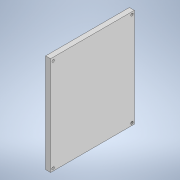
# Autodesk Inventor part: weather_side
Saved by Autodesk Inventor 2021 (Build 250183000, 183)
## iProperties
Created: 2020-04-05
Part Number: weather_side
Material: Generic
Document SubType Name: Modeling
Designer: Daniel
Density: 1 g/cm^3
Appearance: Default
Author: Daniel
Autodesk Inventor part; units mm, degrees
ref_plane "YZ Plane" through (0, 0, 0) normal (1, 0, 0) x (0, 1, 0)
ref_plane "XZ Plane" through (0, 0, 0) normal (0, 1, 0) x (-1, 0, 0)
ref_plane "XY Plane" through (0, 0, 0) normal (0, 0, 1) x (1, 0, 0)
sketch "Sketch1" plane through (0, 0, 0) normal (1, 0, 0) x (0, 1, 0)
  line L0 (0, 0) -> (100, 0)
  line L1 (100, 0) -> (100, -85)
  line L2 (100, -85) -> (0, -85)
  line L3 (0, -85) -> (0, 0)
  dimension "d0" = 100
  dimension "d1" = 85
  dimension "d2" = 100
  constraints: 8 end point, 2 perpendicular, 1 horizontal
  measures "d0" distance of L0.start L0.end
  measures "d1" distance of L0.end L1.end
  measures "d2" distance of L1.end L2.end
extrude "Extrusion1" add sketch "Sketch1" along normal blind 5
sketch "Sketch2" plane through (5, 0, 0) normal (1, 0, 0) x (0, 0, -1)
  line L0 (3.7344, 0) -> (1.2344, 0) construction
  line L1 (0, 0) -> (85, 0) construction
  line L2 (1.2344, 0) -> (1.2344, 2.5) construction
  line L3 (0, 100) -> (0, 0) construction
  line L4 (0, 3.0654) -> (0, 5.5654) construction
  line L5 (0, 5.5654) -> (2.5, 5.5654) construction
  circle A0 centre (2.5, 2.5) radius 1.255
  line L6 (79.4667, 0) -> (79.4667, 2.5) construction
  line L7 (85, 0) -> (85, 100) construction
  line L8 (85, 3.0654) -> (85, 0.5654) construction
  line L9 (85, 0.5654) -> (82.5, 0.5654) construction
  circle A1 centre (82.5, 2.5) radius 1.255 construction
  circle A2 centre (82.5, 2.5) radius 1.255
  line L10 (85, 97.4626) -> (82.5, 97.4626) construction
  line L11 (85, 100) -> (0, 100) construction
  line L12 (81.6079, 100) -> (84.1079, 100) construction
  line L13 (84.1079, 100) -> (84.1079, 97.5) construction
  circle A3 centre (82.5, 97.5) radius 1.25 construction
  circle A4 centre (82.5, 97.5) radius 1.255
  line L14 (0, 96.7939) -> (2.5, 96.7939) construction
  line L15 (2.6492, 100) -> (2.6492, 97.5) construction
  circle A5 centre (2.6492, 96.7939) radius 1.255
  dimension "d5" = 2.5
  dimension "d6" = 2.5
  dimension "d7" = 2.5
  dimension "d8" = 2.5
  dimension "d9" = 2.51
  dimension "d10" = 2.5
  dimension "d11" = 2.5
  dimension "d12" = 2.5
  dimension "d13" = 2.51
  dimension "d14" = 2.51
  dimension "d15" = 2.5
  dimension "d16" = 2.5
  dimension "d17" = 2.5
  dimension "d18" = 2.5
  dimension "d19" = 2.51
  dimension "d20" = 2.5
  dimension "d21" = 2.5
  dimension "d22" = 2.51
  constraints: 24 end point, 11 point on line, 7 perpendicular, 6 centre point, 2 coincident, 1 horizontal
  measures "d5" distance of L0.start L0.end
  measures "d6" distance of L0.end L2.end
  measures "d7" distance of L4.start L4.end
  measures "d8" distance of L4.end L5.end
  measures "d9" diameter of A0
  measures "d10" distance of L6.start L6.end
  measures "d11" distance of L8.start L8.end
  measures "d12" distance of L8.end L9.end
  measures "d13" diameter of A1
  measures "d14" diameter of A2
  measures "d15" distance of L10.start L10.end
  measures "d16" distance of L12.start L12.end
  measures "d17" distance of L12.end L13.end
  measures "d18" diameter of A3
  measures "d19" diameter of A4
  measures "d20" distance of L14.start L14.end
  measures "d21" distance of L15.start L15.end
  measures "d22" diameter of A5
extrude "Extrusion2" cut sketch "Sketch2" against normal blind 4.8
body "Solid1"
